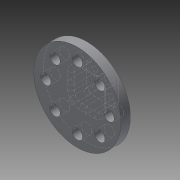
# Autodesk Inventor part: simple_holder_right_angle
Saved by Autodesk Inventor 2013 (Build 170138000, 138)
## iProperties
Created: 2013-03-18
Part Number: simple_holder_right_angle
Material: Generic
Document SubType Name: Modeling
Designer: Mahisorn
Density: 1 g/cm^3
Author: Mahisorn
Autodesk Inventor part; units mm, degrees
ref_plane "YZ Plane" through (0, 0, 0) normal (1, 0, 0) x (0, 1, 0)
ref_plane "XZ Plane" through (0, 0, 0) normal (0, 1, 0) x (-1, 0, 0)
ref_plane "XY Plane" through (0, 0, 0) normal (0, 0, 1) x (1, 0, 0)
sketch "Sketch1" plane through (0, 0, 0) normal (0, 1, 0) x (-1, 0, 0)
  circle A0 centre (0, 0) radius 27.5
  dimension "d0" = 55
  constraints: 1 centre point, 1 coincident
  measures "d0" diameter of A0
extrude "Extrusion1" add sketch "Sketch1" along normal blind 6
sketch "Sketch2" plane through (0, 6, 0) normal (0, 1, 0) x (1, 0, 0)
  circle A0 centre (0, 0) radius 27.5 projected
  point P0 (20, 0)
  point P1 (14.1421, 14.1421)
  point P2 (0, 20)
  point P3 (-14.1421, 14.1421)
  point P4 (-20, 0)
  point P5 (-14.1421, -14.1421)
  point P6 (0, -20)
  point P7 (14.1421, -14.1421)
  dimension "d3" = 20
  dimension "d6" = 360
  constraints: 9 other
  measures "d3" distance of A0.centre point (20, 0)
hole "Hole1" at (20, 6, 0) at (14.1421, 6, -14.1421) at (0, 6, -20) at (-14.1421, 6, -14.1421) at (-20, 6, 0) at (-14.1421, 6, 14.1421) at (0, 6, 20) at (14.1421, 6, 14.1421) direction (0, -1, 0) diameter 6.6 depth 8 tip angle 118 clearance for "Flat Head Machine Screw" size "M6" standard "Ansi Metric M Profile"
sketch "Sketch3" plane through (0, 6, 0) normal (0, 1, 0) x (1, 0, 0)
  circle A0 centre (0, 0) radius 27.5 projected
  line L0 (-5, 10) -> (5, 10)
  line L1 (10, 5) -> (10, -5)
  line L2 (5, -10) -> (-5, -10)
  line L3 (-10, -5) -> (-10, 5)
  arc A1 (-5, 10) -> (-10, 5) centre (-5, 5) ccw
  arc A2 (10, 5) -> (5, 10) centre (5, 5) ccw
  arc A3 (5, -10) -> (10, -5) centre (5, -5) ccw
  arc A4 (-10, -5) -> (-5, -10) centre (-5, -5) ccw
  point P0 (0, 10)
  point P1 (10, 0)
  dimension "d15" = 5
  dimension "d16" = 20
  dimension "d17" = 20
  constraints: 8 end point, 8 point on circle, 8 tangent, 4 centre point, 3 equal radius, 2 midpoint, 2 parallel, 1 horizontal, 1 horizontal alignment, 1 perpendicular, 1 vertical alignment
  measures "d15" radius of A1
  measures "d16" distance between parallel lines of L1 L3
  measures "d17" distance between parallel lines of L2 L0
extrude "Extrusion2" add sketch "Sketch3" along normal blind 10 contours L0 A2 L1 A3 L2 A4 L3 A1
sketch "Sketch4" plane through (0, 16, 0) normal (0, 1, 0) x (1, 0, 0)
  arc A0 (-5, 10) -> (-10, 5) centre (-5, 5) ccw projected
  arc A1 (-10, -5) -> (-5, -10) centre (-5, -5) ccw projected
  arc A2 (5, -10) -> (10, -5) centre (5, -5) ccw projected
  arc A3 (10, 5) -> (5, 10) centre (5, 5) ccw projected
  point P0 (0, 0)
  constraints: 4 coincident
hole "Hole2" at (-5, 16, -5) at (5, 16, -5) at (5, 16, 5) at (-5, 16, 5) direction (0, -1, 0) diameter 3.242 depth 15 tip angle 118 thread size "M4x0.7" class "6H" standard "ANSI Metric M Profile"
fillet "Fillet1" radius 2 8 edges at (8.5355, 6, -8.5355) (10, 6, 0) (8.5355, 6, 8.5355) (0, 6, 10) (-8.5355, 6, 8.5355) (-10, 6, 0) (-8.5355, 6, -8.5355) (0, 6, -10)
body "Solid1"
